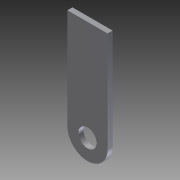
# Autodesk Inventor part: tiltColumnStepperSide
Saved by Autodesk Inventor 2012 (Build 160160000, 160)
## iProperties
Created: 2014-06-13
Part Number: tiltColumnStepperSide
Material: Default
Document SubType Name: Modeling
Designer: Byron
Density: 1 g/cm^3
Author: Byron
Autodesk Inventor part; units mm, degrees
ref_plane "YZ Plane" through (0, 0, 0) normal (1, 0, 0) x (0, 1, 0)
ref_plane "XZ Plane" through (0, 0, 0) normal (0, 1, 0) x (-1, 0, 0)
ref_plane "XY Plane" through (0, 0, 0) normal (0, 0, 1) x (1, 0, 0)
sketch "Sketch1" plane through (0, 0, 0) normal (0, 0, 1) x (1, 0, 0)
  circle A0 centre (106.5872, -122.9172) radius 2.5 projected
  circle A1 centre (106.5872, -122.9172) radius 25.4
  line L0 (81.1872, -122.9172) -> (131.9872, -122.9172)
  line L1 (131.9872, -122.9172) -> (131.9872, 16.7828)
  line L2 (131.9872, 16.7828) -> (81.1872, 16.7828)
  line L3 (81.1872, 16.7828) -> (81.1872, -122.9172)
  circle A2 centre (106.5872, -122.9172) radius 11.5
  point P0 (0, 0)
  point P1 (106.5872, -148.3172)
  dimension "d0" = 50.8
  dimension "d1" = 139.7
  dimension "d4" = 23
  dimension "d9" = 50.8
  constraints: 8 end point, 2 centre point, 2 coincident, 2 parallel, 2 point on circle, 1 horizontal, 1 perpendicular
  measures "d0" diameter of A1
  measures "d1" distance of L1.end L0.end
  measures "d4" diameter of A2
  measures "d9" distance of L1.end L2.end
extrude "Extrusion1" add sketch "Sketch1" against normal blind 6.35 contours L0 A0 | L0 A2 A0 | A0 L0 A2 | A2 L0 A1 | L0 A1 A2 | A1 L3 L2 L1 picked at (105.8251, -122.3305)
sketch "Sketch2" plane through (0, 0, -6.35) normal (0, 0, -1) x (-1, 0, 0)
  arc A0 (-131.9872, -122.9172) -> (-81.1872, -122.9172) centre (-106.5872, -122.9172) ccw projected
  circle A1 centre (-106.5872, -122.9172) radius 11.5
  point P0 (0, 0)
  dimension "d5" = 23
  constraints: 1 centre point, 1 coincident
  measures "d5" diameter of A1
extrude "Extrusion2" cut sketch "Sketch2" against normal through all
sketch "Sketch3" plane through (0, 0, 0) normal (0, 0, 1) x (1, 0, 0)
  circle A0 centre (106.5872, -122.9172) radius 11.5 projected
  arc A1 (81.1872, -122.9172) -> (131.9872, -122.9172) centre (106.5872, -122.9172) ccw projected
  line L0 (131.9872, 16.7828) -> (131.9872, -122.9172) projected
  line L1 (81.1872, 16.7828) -> (131.9872, 16.7828) projected
  line L2 (81.1872, -122.9172) -> (81.1872, 16.7828) projected
  circle A2 centre (122.0872, -107.4172) radius 2 projected
  circle A3 centre (91.0872, -107.4172) radius 2 projected
  circle A4 centre (122.0872, -138.4172) radius 2 projected
  circle A5 centre (91.0872, -138.4172) radius 2 projected
  point P0 (0, 0)
body "Solid1"
